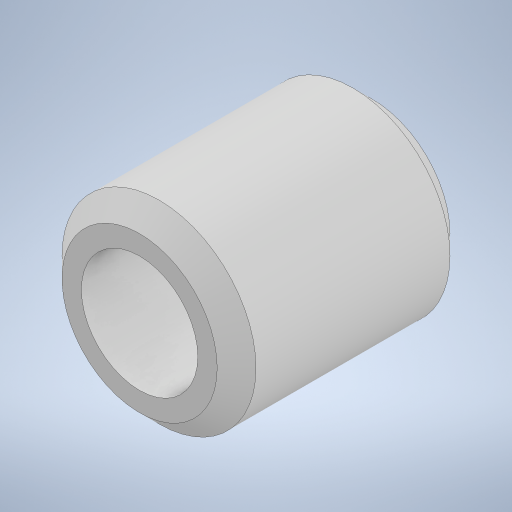
# Autodesk Inventor part: Pieza8-Tarea1
Saved by Autodesk Inventor 2024 (Build 280153000, 153)
## iProperties
Created: 2024-02-16
Part Number: Pieza8-Tarea1
Material: Genérico
Document SubType Name: Modeling
Designer: Diegolap
Density: 1 g/cm^3
Appearance: Valor por defecto
Mass: 2.74836 g
Surface Area: 16.2666 cm^2
Volume: 2.74836 cm^3
Author: Diegolap
Autodesk Inventor part; units mm, degrees
ref_plane "YZ Plane" through (0, 0, 0) normal (1, 0, 0) x (0, 1, 0)
ref_plane "XZ Plane" through (0, 0, 0) normal (0, 1, 0) x (-1, 0, 0)
ref_plane "XY Plane" through (0, 0, 0) normal (0, 0, 1) x (1, 0, 0)
sketch "Boceto1" plane through (0, 0, 0) normal (0, 0, 1) x (1, 0, 0)
  circle A0 centre (0, 0) radius 7.9375
  circle A1 centre (0, 0) radius 4.7625
  dimension "d0" = 15.875
  dimension "d1" = 9.525
  constraints: 2 centre point, 2 coincident
  measures "d0" diameter of A0
  measures "d1" diameter of A1
extrude "Extrusión1" add sketch "Boceto1" along normal blind 19.05 contours A0 | A1
sketch "Boceto2" plane through (0, 0, 19.05) normal (0, 0, 1) x (1, 0, 0)
  circle A0 centre (0, 0) radius 4.7625
  dimension "d4" = 9.525
  constraints: 1 centre point, 1 coincident
  measures "d4" diameter of A0
extrude "Extrusión2" cut sketch "Boceto2" against normal blind 12.7
chamfer "Chaflán1" distance 1.5875 angle 45 1 edges at (-7.9375, 0, 19.05) measured on face at (6.7562, -1.0131, 19.05)
chamfer "Chaflán2" distance 1.5875 angle 45 1 edges at (-7.9375, 0, 0) measured on face at (-0.3189, 2.3213, 0)
sketch "Boceto3" plane through (0, 0, 0) normal (0, 0, -1) x (-1, 0, 0)
  point P0 (0, 0)
